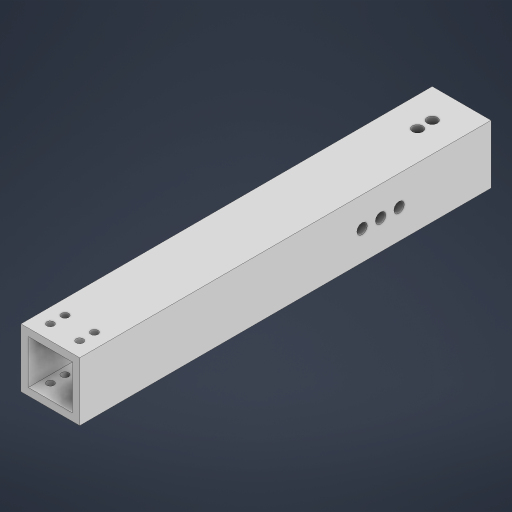
# Autodesk Inventor part: CS_Climb_Inner_Tube
Saved by Autodesk Inventor 2023 (Build 270158000, 158)
## iProperties
Created: 2024-02-19
Part Number: CS_Climb_Inner_Tube
Material: Generic
Document SubType Name: Modeling
Designer: kelle
Density: 1 g/cm^3
Appearance: Default
Author: kelle
Autodesk Inventor part; units mm, degrees
ref_plane "YZ Plane" through (0, 0, 0) normal (1, 0, 0) x (0, 1, 0)
ref_plane "XZ Plane" through (0, 0, 0) normal (0, 1, 0) x (-1, 0, 0)
ref_plane "XY Plane" through (0, 0, 0) normal (0, 0, 1) x (1, 0, 0)
sketch "Sketch1" plane through (0, 0, 0) normal (0, 0, 1) x (1, 0, 0)
  line L0 (12.7, -12.7) -> (-12.7, -12.7)
  line L1 (-12.7, -12.7) -> (-12.7, 12.7)
  line L2 (-12.7, 12.7) -> (12.7, 12.7)
  line L3 (12.7, 12.7) -> (12.7, -12.7)
  line L4 (12.7, -12.7) -> (-12.7, 12.7) construction
  line L5 (-12.7, -12.7) -> (12.7, 12.7) construction
  line L6 (9.525, 9.525) -> (-9.525, 9.525)
  line L7 (-9.525, 9.525) -> (-9.525, -9.525)
  line L8 (-9.525, -9.525) -> (9.525, -9.525)
  line L9 (9.525, -9.525) -> (9.525, 9.525)
  point P0 (0, 0)
  dimension "d0" = 25.4
  dimension "d1" = 25.4
  dimension "d2" = 3.175
  constraints: 20 end point, 4 parallel, 2 midpoint, 2 perpendicular, 1 horizontal, 3 other
  measures "d0" distance of L1.end L2.end
  measures "d1" distance of L0.end L1.end
  measures "d2" distance between parallel lines of L2 L6
extrude "Extrusion1" add sketch "Sketch1" along normal blind 177.8
sketch "Sketch2" plane through (12.7, -12.7, 0) normal (1, 0, 0) x (0, 0, -1)
  line L0 (0, 0) -> (0, 25.4) construction
  line L1 (0, 25.4) -> (-177.8, 25.4) construction
  line L2 (-177.8, 0) -> (-177.8, 25.4) construction
  line L3 (0, 0) -> (-177.8, 0) construction
  line L4 (-177.8, 22.225) -> (-177.8, 3.175) construction
  line L5 (-177.8, 12.7) -> (0, 12.7) construction
  line L6 (-31.75, 25.4) -> (-31.75, 0) construction
  circle A0 centre (-39.75, 12.7) radius 2.25
  circle A1 centre (-47.75, 12.7) radius 2.25
  circle A2 centre (-55.75, 12.7) radius 2.25
  dimension "d5" = 31.75
  dimension "d6" = 4.5
  dimension "d7" = 8
  dimension "d8" = 4.5
  dimension "d9" = 8
  dimension "d10" = 4.5
  dimension "d11" = 8
  constraints: 5 point on line, 4 end point, 3 centre point, 1 horizontal, 1 midpoint, 1 perpendicular
  measures "d5" distance between parallel lines of L0 L6
  measures "d6" diameter of A0
  measures "d7" distance from line of L6 A0.centre
  measures "d8" diameter of A1
  measures "d9" distance of A0.centre A1.centre
  measures "d10" diameter of A2
  measures "d11" distance of A1.centre A2.centre
extrude "Extrusion2" cut sketch "Sketch2" against normal through all
sketch "Sketch3" plane through (-12.7, 12.7, 0) normal (0, 1, 0) x (1, 0, 0)
  line L0 (12.7, 0) -> (12.7, -177.7213) construction
  circle A0 centre (12.7, -12.7) radius 2.25
  circle A1 centre (12.7, -19.05) radius 2.25
  line L1 (25.4, 0) -> (0, 0) projected
  dimension "d14" = 4.5
  dimension "d15" = 4.5
  dimension "d16" = 12.7
  dimension "d17" = 6.35
  constraints: 2 centre point, 2 end point, 2 point on line, 1 vertical
  measures "d14" diameter of A0
  measures "d15" diameter of A1
  measures "d16" distance from line of L1 A0.centre
  measures "d17" distance of A1.centre A0.centre
extrude "Extrusion3" cut sketch "Sketch3" against normal blind 25.4
sketch "Sketch4" plane through (-12.7, 12.7, 0) normal (0, 1, 0) x (1, 0, 0)
  line L0 (12.7, 0) -> (12.7, -177.8) construction
  line L1 (3.175, -177.8) -> (22.225, -177.8) construction
  circle A0 centre (6.35, -171.45) radius 1.5875
  line L2 (0, 0) -> (0, -177.8) projected
  circle A1 centre (19.05, -171.45) radius 1.5875
  line L3 (25.4, 0) -> (25.4, -177.8) projected
  circle A2 centre (6.35, -165.1) radius 1.5875
  circle A3 centre (19.05, -165.1) radius 1.5875
  dimension "d20" = 3.175
  dimension "d21" = 6.35
  dimension "d22" = 6.35
  dimension "d23" = 3.175
  dimension "d24" = 6.35
  dimension "d25" = 6.35
  dimension "d26" = 3.175
  dimension "d27" = 6.35
  dimension "d28" = 6.35
  dimension "d29" = 3.175
  dimension "d30" = 6.35
  dimension "d31" = 6.35
  constraints: 4 centre point, 2 end point, 1 midpoint
  measures "d20" diameter of A0
  measures "d21" distance from line of L1 A0.centre
  measures "d22" distance from line of L2 A0.centre
  measures "d23" diameter of A1
  measures "d24" distance from line of L1 A1.centre
  measures "d25" distance from line of L3 A1.centre
  measures "d26" diameter of A2
  measures "d27" distance of A0.centre A2.centre
  measures "d28" distance from line of L2 A2.centre
  measures "d29" diameter of A3
  measures "d30" distance from line of L3 A3.centre
  measures "d31" distance of A1.centre A3.centre
extrude "Extrusion4" cut sketch "Sketch4" against normal through all
body "Solid1"
